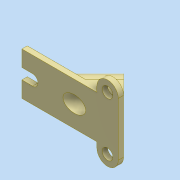
# Autodesk Inventor part: BT2
Saved by Autodesk Inventor 2016 (Build 200138000, 138)
## iProperties
Created: 2016-08-16
Part Number: BT2
Material: Nylon 6/6
Document SubType Name: Modeling
Designer: ADMIN
Density: 1.13 g/cm^3
Appearance: Nylon 6
Author: ADMIN
Autodesk Inventor part; units mm, degrees
ref_plane "YZ Plane" through (0, 0, 0) normal (1, 0, 0) x (0, 1, 0)
ref_plane "XZ Plane" through (0, 0, 0) normal (0, 1, 0) x (-1, 0, 0)
sketch "Sketch1" plane through (0, 0, 0) normal (0, 1, 0) x (-1, 0, 0)
  line L0 (-40, 0) -> (-40, -100)
  line L1 (-30, -100) -> (-10, -100)
  line L2 (0, -10) -> (140, -10)
  line L3 (140, -90) -> (0, -90)
  arc A0 (0, 0) -> (-40, 0) centre (-20, 0) ccw
  arc A1 (-40, -100) -> (0, -100) centre (-20, -100) ccw
  circle A2 centre (-20, 0) radius 10
  circle A3 centre (-20, -100) radius 10
  arc A4 (120, -40) -> (120, -60) centre (120, -50) ccw
  line L4 (120, -40) -> (140, -40)
  line L5 (120, -60) -> (140, -60)
  line L6 (140, -10) -> (140, -40)
  line L7 (140, -60) -> (140, -90)
  line L8 (0, -100) -> (0, -90)
  line L9 (0, -10) -> (0, 0)
  line L10 (-30, 0) -> (-40, 0)
  dimension "d4" = 20
  dimension "d0" = 40
  dimension "d1" = 100
  dimension "d2" = 140
  dimension "d3" = 80
  dimension "d5" = 20
  dimension "d6" = 20
  dimension "d8" = 20
  dimension "d9" = 20
  constraints: 22 end point, 8 point on circle, 4 centre point, 4 parallel, 3 perpendicular, 2 coincident, 2 horizontal, 1 horizontal alignment, 1 midpoint, 2 other
  measures "d0" distance of L8.start L0.end
  measures "d1" distance of L0.end L0.start
  measures "d2" distance of L3.start L3.end
  measures "d3" distance of L2.end L3.start
  measures "d5" diameter of A3
  measures "d6" diameter of A4
  measures "d8" distance of L4.start L4.end
  measures "d9" distance of L5.start L5.end
extrude "Extrusion1" add sketch "Sketch1" along normal blind 10
ref_plane "Work Plane1" through (40, 10, 0) normal (0.7071, 0.7071, 0) x (0, 0, -1)
sketch "Sketch2" plane through (0, 10, 0) normal (0, 1, 0) x (1, 0, 0)
  point P0 (0, 0)
sketch "Sketch3" plane through (40, 10, 0) normal (0.7071, 0.7071, 0) x (0, 0, -1)
  line L0 (90, 51) -> (90, 0)
  line L1 (90, 0) -> (10, 0)
  line L2 (10, 0) -> (10, 51)
  arc A0 (90, 51) -> (10, 51) centre (50, 51) ccw
  circle A1 centre (50, 51) radius 15
  point P0 (0, 21.2132)
  point P1 (90, 28.2843)
  dimension "d13" = 51
  dimension "d14" = 30
  constraints: 6 end point, 2 centre point, 2 point on circle, 1 coincident, 1 parallel
  measures "d13" distance of L1.end L2.end
  measures "d14" diameter of A1
extrude "Extrusion2" add sketch "Sketch3" against normal up to next
sketch "Sketch4" plane through (40, 10, 0) normal (0.7071, 0.7071, 0) x (0, 0, -1)
  circle A0 centre (50, 51) radius 15 projected
  circle A1 centre (50, 51) radius 15
  point P0 (0, 21.2132)
  dimension "d17" = 30
  constraints: 1 centre point, 1 coincident
  measures "d17" diameter of A1
extrude "Extrusion3" cut sketch "Sketch4" against normal up to surface surface through (-48.5464, 0, -50) normal (0, 1, 0)
body "Solid1"
